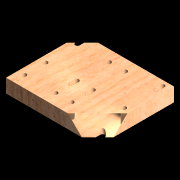
# Autodesk Inventor part: AXYZB
Saved by Autodesk Inventor 2016 (Build 200138000, 138)
## iProperties
Created: 2015-08-05
Part Number: AXYZB
Material: PC/ABS Plastic
Document SubType Name: Modeling
Designer: Jose
Density: 0.357273 g/cm^3
Appearance: Smooth - White
Mass: 113.976 g
Surface Area: 367.474 cm^2
Volume: 207.23 cm^3
Author: Jose
Autodesk Inventor part; units mm, degrees
ref_plane "YZ Plane" through (0, 0, 0) normal (1, 0, 0) x (0, 1, 0)
ref_plane "XZ Plane" through (0, 0, 0) normal (0, 1, 0) x (-1, 0, 0)
ref_plane "XY Plane" through (0, 0, 0) normal (0, 0, 1) x (1, 0, 0)
sketch "Sketch1" plane through (0, 0, 0) normal (0, 0, 1) x (1, 0, 0)
  circle A0 centre (101.375, -25.0526) radius 3.05 projected
  circle A1 centre (-2.375, -39.3026) radius 3.05 projected
  circle A2 centre (101.375, -39.3026) radius 3.05 projected
  circle A3 centre (-2.375, -25.0526) radius 3.05 projected
  circle A4 centre (59.875, 2.8224) radius 3.05 projected
  circle A5 centre (39.125, 2.8224) radius 3.05 projected
  circle A6 centre (39.125, -67.1776) radius 3.05 projected
  circle A7 centre (59.875, -67.1776) radius 3.05 projected
  line L0 (109.5, 17.8224) -> (-10.5, 17.8224) projected
  line L1 (-10.5, 17.8224) -> (-10.5, -82.1776) projected
  line L2 (-10.5, -82.1776) -> (109.5, -82.1776) projected
  line L3 (109.5, -82.1776) -> (109.5, 17.8224) projected
  arc A8 (36.075, -25.0526) -> (42.175, -25.0526) centre (39.125, -25.0526) ccw projected
  arc A9 (62.925, -39.3026) -> (56.825, -39.3026) centre (59.875, -39.3026) ccw projected
  arc A10 (42.175, -39.3026) -> (36.075, -39.3026) centre (39.125, -39.3026) ccw projected
  arc A11 (56.825, -25.0526) -> (62.925, -25.0526) centre (59.875, -25.0526) ccw projected
  arc A12 (-5.425, 2.8224) -> (0.675, 2.8224) centre (-2.375, 2.8224) ccw projected
  arc A13 (98.325, 2.8224) -> (104.425, 2.8224) centre (101.375, 2.8224) ccw projected
  arc A14 (104.425, -67.1776) -> (98.325, -67.1776) centre (101.375, -67.1776) ccw projected
  arc A15 (0.675, -67.1776) -> (-5.425, -67.1776) centre (-2.375, -67.1776) ccw projected
  line L4 (0.675, -67.1776) -> (0.675, -75.1776) projected
  arc A16 (-5.425, -75.1776) -> (0.675, -75.1776) centre (-2.375, -75.1776) ccw projected
  line L5 (-5.425, -75.1776) -> (-5.425, -67.1776) projected
  line L6 (104.425, -67.1776) -> (104.425, -75.1776) projected
  arc A17 (98.325, -75.1776) -> (104.425, -75.1776) centre (101.375, -75.1776) ccw projected
  line L7 (98.325, -75.1776) -> (98.325, -67.1776) projected
  line L8 (-5.425, 2.8224) -> (-5.425, 10.8224) projected
  arc A18 (0.675, 10.8224) -> (-5.425, 10.8224) centre (-2.375, 10.8224) ccw projected
  line L9 (0.675, 10.8224) -> (0.675, 2.8224) projected
  line L10 (42.175, -39.3026) -> (42.175, -47.3026) projected
  arc A19 (36.075, -47.3026) -> (42.175, -47.3026) centre (39.125, -47.3026) ccw projected
  line L11 (36.075, -47.3026) -> (36.075, -39.3026) projected
  line L12 (62.925, -39.3026) -> (62.925, -47.3026) projected
  arc A20 (56.825, -47.3026) -> (62.925, -47.3026) centre (59.875, -47.3026) ccw projected
  line L13 (56.825, -47.3026) -> (56.825, -39.3026) projected
  line L14 (62.925, -17.0526) -> (62.925, -25.0526) projected
  line L15 (56.825, -25.0526) -> (56.825, -17.0526) projected
  arc A21 (62.925, -17.0526) -> (56.825, -17.0526) centre (59.875, -17.0526) ccw projected
  line L16 (104.425, 10.8224) -> (104.425, 2.8224) projected
  line L17 (98.325, 2.8224) -> (98.325, 10.8224) projected
  arc A22 (104.425, 10.8224) -> (98.325, 10.8224) centre (101.375, 10.8224) ccw projected
  line L18 (42.175, -17.0526) -> (42.175, -25.0526) projected
  line L19 (36.075, -25.0526) -> (36.075, -17.0526) projected
  arc A23 (42.175, -17.0526) -> (36.075, -17.0526) centre (39.125, -17.0526) ccw projected
  point P0 (0, 0)
  point P1 (39.5, -24.775)
  point P2 (60.5, -39.025)
  point P3 (39.5, -39.025)
  point P4 (60.5, -24.775)
  point P5 (-1.375, 3.1)
  point P6 (101.375, 3.1)
  point P7 (101.375, -66.9)
  point P8 (-1.375, -66.9)
extrude "Extrusion1" add sketch "Sketch1" along normal blind 18
sketch "Sketch2" plane through (0, 0, 18) normal (0, 0, 1) x (1, 0, 0)
  arc A0 (0.675, -67.1776) -> (-5.425, -67.1776) centre (-2.375, -67.1776) ccw projected
  line L0 (0.675, -67.1776) -> (0.675, -75.1776) projected
  arc A1 (-5.425, -75.1776) -> (0.675, -75.1776) centre (-2.375, -75.1776) ccw projected
  line L1 (-5.425, -75.1776) -> (-5.425, -67.1776) projected
  arc A2 (104.425, -67.1776) -> (98.325, -67.1776) centre (101.375, -67.1776) ccw projected
  line L2 (104.425, -67.1776) -> (104.425, -75.1776) projected
  arc A3 (98.325, -75.1776) -> (104.425, -75.1776) centre (101.375, -75.1776) ccw projected
  line L3 (98.325, -75.1776) -> (98.325, -67.1776) projected
  arc A4 (98.325, 2.8224) -> (104.425, 2.8224) centre (101.375, 2.8224) ccw projected
  line L4 (98.325, 2.8224) -> (98.325, 10.8224) projected
  arc A5 (104.425, 10.8224) -> (98.325, 10.8224) centre (101.375, 10.8224) ccw projected
  line L5 (104.425, 10.8224) -> (104.425, 2.8224) projected
  arc A6 (-5.425, 2.8224) -> (0.675, 2.8224) centre (-2.375, 2.8224) ccw projected
  line L6 (-5.425, 2.8224) -> (-5.425, 10.8224) projected
  arc A7 (0.675, 10.8224) -> (-5.425, 10.8224) centre (-2.375, 10.8224) ccw projected
  line L7 (0.675, 10.8224) -> (0.675, 2.8224) projected
  arc A8 (56.825, -25.0526) -> (62.925, -25.0526) centre (59.875, -25.0526) ccw projected
  line L8 (56.825, -25.0526) -> (56.825, -17.0526) projected
  arc A9 (62.925, -17.0526) -> (56.825, -17.0526) centre (59.875, -17.0526) ccw projected
  line L9 (62.925, -17.0526) -> (62.925, -25.0526) projected
  arc A10 (42.175, -39.3026) -> (36.075, -39.3026) centre (39.125, -39.3026) ccw projected
  line L10 (42.175, -39.3026) -> (42.175, -47.3026) projected
  arc A11 (36.075, -47.3026) -> (42.175, -47.3026) centre (39.125, -47.3026) ccw projected
  line L11 (36.075, -47.3026) -> (36.075, -39.3026) projected
  arc A12 (62.925, -39.3026) -> (56.825, -39.3026) centre (59.875, -39.3026) ccw projected
  line L12 (62.925, -39.3026) -> (62.925, -47.3026) projected
  arc A13 (56.825, -47.3026) -> (62.925, -47.3026) centre (59.875, -47.3026) ccw projected
  line L13 (56.825, -47.3026) -> (56.825, -39.3026) projected
  arc A14 (36.075, -25.0526) -> (42.175, -25.0526) centre (39.125, -25.0526) ccw projected
  line L14 (36.075, -25.0526) -> (36.075, -17.0526) projected
  arc A15 (42.175, -17.0526) -> (36.075, -17.0526) centre (39.125, -17.0526) ccw projected
  line L15 (42.175, -17.0526) -> (42.175, -25.0526) projected
  circle A16 centre (59.875, -67.1776) radius 3.05 projected
  circle A17 centre (39.125, -67.1776) radius 3.05 projected
  circle A18 centre (39.125, 2.8224) radius 3.05 projected
  circle A19 centre (59.875, 2.8224) radius 3.05 projected
  circle A20 centre (-2.375, -25.0526) radius 3.05 projected
  circle A21 centre (101.375, -39.3026) radius 3.05 projected
  circle A22 centre (-2.375, -39.3026) radius 3.05 projected
  circle A23 centre (101.375, -25.0526) radius 3.05 projected
  line L16 (109.5, 17.8224) -> (-10.5, 17.8224) projected
  line L17 (-10.5, 17.8224) -> (-10.5, -82.1776) projected
  line L18 (-10.5, -82.1776) -> (109.5, -82.1776) projected
  line L19 (109.5, -82.1776) -> (109.5, 17.8224) projected
  point P0 (0, 0)
extrude "Extrusion2" add sketch "Sketch2" against normal blind 18 contours L8 A9 L9 A8 | L14 A15 L15 A14 | A20 | A23
body "Solid1"
